Autodesk Fusion 360 part; units mm, degrees
note: some values were not read from the file. Chosen so that the rebuilt part matches the saved one: which face or edge a step refers to.
(part 2 of 2)
sketch "Sketch63" plane through (0, 0, -22) normal (0, 0, 1) x (-1, 0, 0)
  line L0 (-15, -20.0531) -> (-15, -15)
  line L1 (-15, -15) -> (-65, -15)
  line L2 (-65, -15) -> (-65, -0.5084)
  circle A0 centre (-69.7753, -0.5084) radius 4.7753
  line L3 (-65, -0.5084) -> (-65, 13.9831)
  line L4 (-65, 13.9831) -> (-82.6499, 13.9831)
  line L5 (-82.6499, 13.9831) -> (-96.6499, -0.0169)
  line L6 (-96.6499, -0.0169) -> (-96.6499, -72.0837)
  line L7 (-96.6499, -72.0837) -> (-82.6499, -86.0837)
  line L8 (-82.6499, -86.0837) -> (-65, -86.0837)
  line L9 (-65, -86.0837) -> (-65, -71.5419)
  circle A1 centre (-69.9244, -71.5419) radius 4.9244
  line L10 (-65, -71.5419) -> (-65, -57)
  line L11 (-65, -57) -> (-15, -57)
  line L12 (-15, -57) -> (-15, -52)
  line L13 (-15, -52) -> (-18, -52)
  line L14 (-18, -52) -> (-18, -20.0531)
  line L15 (-18, -20.0531) -> (-15, -20.0531)
  circle A2 centre (-85.0223, -71.5419) radius 5
  circle A3 centre (-84.8815, -0.5084) radius 5
  dimension "d174" = 10
  dimension "d175" = 10
  measures "d174" diameter of A2
  measures "d175" diameter of A3
extrude "Extrude63" cut sketch "Sketch63" against normal blind 10 contours A2 | A3 bodies 24
sketch "Sketch64" plane through (0, 0, -22) normal (0, 0, 1) x (-1, 0, 0)
  circle A0 centre (-85.0223, -71.5419) radius 5
  circle A1 centre (-84.8815, -0.5084) radius 5
  line L0 (-15, -20.0531) -> (-15, -15)
  line L1 (-15, -15) -> (-65, -15)
  line L2 (-65, -15) -> (-65, -0.5084)
  circle A2 centre (-69.7753, -0.5084) radius 4.7753
  line L3 (-65, -0.5084) -> (-65, 13.9831)
  line L4 (-65, 13.9831) -> (-82.6499, 13.9831)
  line L5 (-82.6499, 13.9831) -> (-96.6499, -0.0169)
  line L6 (-96.6499, -0.0169) -> (-96.6499, -72.0837)
  line L7 (-96.6499, -72.0837) -> (-82.6499, -86.0837)
  line L8 (-82.6499, -86.0837) -> (-65, -86.0837)
  line L9 (-65, -86.0837) -> (-65, -71.5419)
  circle A3 centre (-69.9244, -71.5419) radius 4.9244
  line L10 (-65, -71.5419) -> (-65, -57)
  line L11 (-65, -57) -> (-15, -57)
  line L12 (-15, -57) -> (-15, -52)
  line L13 (-15, -52) -> (-18, -52)
  line L14 (-18, -52) -> (-18, -20.0531)
  line L15 (-18, -20.0531) -> (-15, -20.0531)
  line L16 (-96.6499, -49.9799) -> (-91, -49.9799)
  line L17 (-91, -49.9799) -> (-91, -20)
  line L18 (-91, -20) -> (-96.6499, -20)
  line L19 (-96.6499, -20) -> (-96.6499, -49.9799)
  line L20 (-65, -86.0837) -> (-65, -84)
  line L21 (-65, -84) -> (-82, -84)
  line L22 (-82, -84) -> (-95, -72)
  line L23 (-95, -72) -> (-95, 0)
  line L24 (-95, 0) -> (-82, 12)
  line L25 (-82, 12) -> (-65, 12)
  constraint horizontal L16
  constraint vertical L17
  constraint horizontal L18
  constraint vertical L19
  constraint coincident L6 L16.start
  constraint coincident L8.end L9.start
  constraint coincident L9 L20.end
  constraint perpendicular L8 L20
  constraint perpendicular L20 L21
  constraint perpendicular L16 L23
  constraint coincident L3 L25.end
  constraint perpendicular L3 L25
extrude "Extrude64" add sketch "Sketch64" along normal blind 24 separate body contours L3 L4 L5 L6 L18 L23 L24 L25 | L6 L16 L18 L19 L23 | L6 L7 L8 L9 L16 L20 L21 L22 L23 makes body 26
extrude "Extrude65" cut 1 faces at (76.55, 85.3892, 2) along direction (0, 0, -1) blind 2 on bodies 26 bodies 10 26
extrude "Extrude66" cut 1 faces at (76.55, 85.3892, 0) along direction (0, 0, -1) blind 1 on bodies 26 bodies 26
sketch "Sketch65" plane through (0, 0, 6.5) normal (0, 0, 1) x (-1, 0, 0)
  line L0 (-75, -10) -> (-75, -12)
  line L1 (-75, -12) -> (-75, -60)
  line L2 (-75, -60) -> (-75, -62)
  line L3 (-75, -62) -> (-95, -62)
  line L4 (-95, -62) -> (-95, -72)
  line L5 (-95, -72) -> (-83, -84)
  line L6 (-83, -84) -> (-65, -84)
  line L7 (-65, -84) -> (-65, -57)
  line L8 (-65, -57) -> (-26, -57)
  line L9 (-26, -57) -> (-26, -15)
  line L10 (-26, -15) -> (-65, -15)
  line L11 (-65, -15) -> (-65, 12)
  line L12 (-65, 12) -> (-83, 12)
  line L13 (-83, 12) -> (-95, 0)
  line L14 (-95, 0) -> (-95, -10)
  line L15 (-95, -10) -> (-75, -10)
  circle A0 centre (-69.7753, -0.5084) radius 1.5
  circle A1 centre (-69.9244, -71.5419) radius 1.5
  circle A2 centre (-90, -70) radius 2.5
  circle A3 centre (-90, -2) radius 2.5
  circle A4 centre (-81, -70) radius 2
  circle A5 centre (-81, -2) radius 2
  dimension "d184" = 5
  dimension "d185" = 5
  dimension "d186" = 4
  dimension "d187" = 4
  measures "d184" diameter of A2
  measures "d185" diameter of A3
  measures "d186" diameter of A4
  measures "d187" diameter of A5
extrude "Extrude67" cut sketch "Sketch65" against normal blind 3 contours A2 | A3 | A4 | A5 bodies 25
sketch "Sketch66" plane through (0, 0, -1) normal (0, 0, 1) x (-1, 0, 0)
  line L0 (-82, 12) -> (-65, 12)
  line L1 (-65, 12) -> (-65, 13.9831)
  line L2 (-65, 13.9831) -> (-82.6499, 13.9831)
  line L3 (-82.6499, 13.9831) -> (-96.6499, -0.0169)
  line L4 (-96.6499, -0.0169) -> (-96.6499, -72.0837)
  line L5 (-96.6499, -72.0837) -> (-82.6499, -86.0837)
  line L6 (-82.6499, -86.0837) -> (-65, -86.0837)
  line L7 (-65, -86.0837) -> (-65, -84)
  line L8 (-65, -84) -> (-82, -84)
  line L9 (-82, -84) -> (-95, -72)
  line L10 (-95, -72) -> (-95, 0)
  line L11 (-95, 0) -> (-82, 12)
  line L12 (-96.6499, -60.0117) -> (-95, -60.0117)
  line L13 (-95, -60.0117) -> (-95, -12)
  line L14 (-95, -12) -> (-96.6499, -12)
  line L15 (-96.6499, -12) -> (-96.6499, -60.0117)
  constraint horizontal L12
  constraint vertical L13
  constraint horizontal L14
  constraint vertical L15
  constraint coincident L10 L13.end
  constraint coincident L4 L12.start
extrude "Extrude68" add sketch "Sketch66" along normal blind 5 contours L0 L1 L2 L3 L4 L10 L11 L14 | L4 L5 L6 L7 L8 L9 L10 L12 bodies 26
sketch "Sketch67" plane through (0, 0, -22) normal (0, 0, 1) x (-1, 0, 0)
  circle A0 centre (-85.0223, -71.5419) radius 5
  circle A1 centre (-84.8815, -0.5084) radius 5
  line L0 (-15, -20.0531) -> (-15, -15)
  line L1 (-15, -15) -> (-65, -15)
  line L2 (-65, -15) -> (-65, -0.5084)
  circle A2 centre (-69.7753, -0.5084) radius 4.7753
  line L3 (-65, -0.5084) -> (-65, 13.9831)
  line L4 (-65, 13.9831) -> (-82.6499, 13.9831)
  line L5 (-82.6499, 13.9831) -> (-96.6499, -0.0169)
  line L6 (-96.6499, -0.0169) -> (-96.6499, -72.0837)
  line L7 (-96.6499, -72.0837) -> (-82.6499, -86.0837)
  line L8 (-82.6499, -86.0837) -> (-65, -86.0837)
  line L9 (-65, -86.0837) -> (-65, -71.5419)
  circle A3 centre (-69.9244, -71.5419) radius 4.9244
  line L10 (-65, -71.5419) -> (-65, -57)
  line L11 (-65, -57) -> (-15, -57)
  line L12 (-15, -57) -> (-15, -52)
  line L13 (-15, -52) -> (-18, -52)
  line L14 (-18, -52) -> (-18, -20.0531)
  line L15 (-18, -20.0531) -> (-15, -20.0531)
  line L16 (-95, -50) -> (-90, -50)
  line L17 (-90, -50) -> (-90, -20)
  line L18 (-90, -20) -> (-95, -20)
  line L19 (-95, -20) -> (-95, -50)
  constraint horizontal L16
  constraint vertical L17
  constraint horizontal L18
  constraint vertical L19
extrude "Extrude69" add sketch "Sketch67" along normal blind 10 contours L16 L17 L18 L19 bodies 24
sketch "Sketch68" plane through (95, 0, 0) normal (1, 0, 0) x (0, 1, 0)
  line L0 (20, -22) -> (50, -22)
  line L1 (50, -22) -> (50, -12)
  line L2 (50, -12) -> (20, -12)
  line L3 (20, -12) -> (20, -22)
  circle A0 centre (45, -17) radius 1.5
  circle A1 centre (25, -17) radius 1.5
  dimension "d194" = 3
  dimension "d195" = 3
  measures "d194" diameter of A0
  measures "d195" diameter of A1
extrude "Extrude70" cut sketch "Sketch68" against normal blind 10 contours A0 | A1 bodies 24
extrude "Extrude71" cut sketch "Sketch68" along normal blind 4 contours A0 | A1 bodies 26
extrude "Extrude72" add 2 faces at (76.55, 85.3892, 4) (76.55, -13.3221, 4) along direction (0, 0, 1) blind 1 on bodies 26 bodies 26
extrude "Extrude73" cut 2 faces at (96, 49.7337, 4.7398) (96, 25.3431, 3.7629) along direction (-1, 0, 0) blind 12 on bodies 10 bodies 10
extrude "Extrude74" cut 2 faces at (95, 24.4418, 1.8385) (95, 49.4418, 1.8385) along direction (-1, 0, 0) blind 11 on bodies 10 bodies 10
sketch "Sketch69" plane through (84, 0, 0) normal (1, 0, 0) x (0, 1, 0)
  line L0 (58.5, 19) -> (13.5, 19)
  line L1 (13.5, 19) -> (13.5, -1)
  line L2 (13.5, -1) -> (58.5, -1)
  line L3 (58.5, -1) -> (58.5, 19)
  circle A0 centre (49.9081, 9) radius 8
  circle A1 centre (21.9658, 9) radius 8
  dimension "d206" = 16
  dimension "d207" = 16
  measures "d206" diameter of A0
  measures "d207" diameter of A1
extrude "Extrude75" add sketch "Sketch69" along normal blind 12 contours A0 | A1 bodies 10
sketch "Sketch70" plane through (95, 0, 0) normal (1, 0, 0) x (0, 1, 0)
  circle A0 centre (45, -17) radius 1.5
  circle A1 centre (25, -17) radius 1.5
  line L0 (20, -22) -> (50, -22)
  line L1 (50, -22) -> (50, -12)
  line L2 (50, -12) -> (20, -12)
  line L3 (20, -12) -> (20, -22)
  line L4 (50, -12) -> (58.5, -1)
  line L5 (58.5, -1) -> (58.5, 19)
  line L6 (58.5, 19) -> (13.5, 19)
  line L7 (13.5, 19) -> (13.5, -1)
  line L8 (13.5, -1) -> (20, -12)
  constraint coincident L1.end L2.start
  constraint perpendicular L2 L5
  constraint perpendicular L5 L6
  constraint perpendicular L6 L7
  constraint coincident L2.end L3.start
sketch "Sketch71" plane through (96, 0, 0) normal (1, 0, 0) x (0, 1, 0)
  circle A0 centre (21.9658, 9) radius 8
  circle A1 centre (21.9658, 9) radius 8
  constraint concentric A0 A1
sketch "Sketch72" plane through (96, 0, 0) normal (1, 0, 0) x (0, 1, 0)
  circle A0 centre (49.9081, 9) radius 8
  circle A1 centre (49.9081, 9) radius 8
  constraint concentric A0 A1
extrude "Extrude76" add sketch "Sketch70" against normal blind 1.5 contours L2 L4 L5 L6 L7 L8 bodies 24
extrude "Extrude77" cut sketch "Sketch72" sketch "Sketch71" against normal blind 3 of sketch 2 bodies 24
sketch "Sketch73" plane through (0, 86, 0) normal (0, 1, 0) x (-1, 0, 0)
  circle A0 centre (-29.5, -11) radius 2.5
  circle A1 centre (-29.5, -11) radius 33
extrude "Extrude78" add 2 faces at (88.8333, 60.6667, 20.5) (88.8333, 11.3333, 20.5) along direction (0, 0, 1) blind 1 on bodies 25 bodies 25
sketch "Sketch74" plane through (0, 86, 0) normal (0, 1, 0) x (-1, 0, 0)
sketch "Sketch75" plane through (0, 0, -23.5) normal (0, 0, -1) x (1, 0, 0)
  circle A0 centre (85.0223, -71.5419) radius 5
  circle A1 centre (84.8815, -0.5084) radius 5
  circle A2 centre (69.9244, -71.5419) radius 1.5
  circle A3 centre (69.7753, -0.5084) radius 1.5
  line L0 (1, -20.0531) -> (18, -20.0531)
  line L1 (18, -20.0531) -> (18, -52)
  line L2 (18, -52) -> (1, -52)
  line L3 (1, -52) -> (1, -57)
  line L4 (1, -57) -> (65, -57)
  line L5 (65, -57) -> (65, -86.0837)
  line L6 (65, -86.0837) -> (82.6499, -86.0837)
  line L7 (82.6499, -86.0837) -> (96.6499, -72.0837)
  line L8 (96.6499, -72.0837) -> (96.6499, -0.0169)
  line L9 (96.6499, -0.0169) -> (82.6499, 13.9831)
  line L10 (82.6499, 13.9831) -> (65, 13.9831)
  line L11 (65, 13.9831) -> (65, -15)
  line L12 (65, -15) -> (1, -15)
  line L13 (1, -15) -> (1, -20.0531)
  circle A4 centre (75, -65) radius 5
  circle A5 centre (75, -7.0195) radius 5
  dimension "d216" = 10
  measures "d216" diameter of A5
extrude "Extrude79" add sketch "Sketch75" along normal blind 28 separate body contours A4 | A5 makes body 27 at (79.9752, 65.4978, -42.1667) makes body 28 at (79.9752, 7.5173, -42.1667)
sketch "Sketch76" plane through (0, 0, -51.5) normal (0, 0, -1) x (1, 0, 0)
  circle A0 centre (75, -65) radius 5
  circle A1 centre (75, -65) radius 1.5
  dimension "d219" = 3
  constraint concentric A0 A1
  measures "d219" diameter of A1
sketch "Sketch77" plane through (0, 0, -51.5) normal (0, 0, -1) x (1, 0, 0)
  circle A0 centre (75, -7.0195) radius 5
  circle A1 centre (75, -7.0195) radius 1.5
  dimension "d220" = 3
  constraint concentric A0 A1
  measures "d220" diameter of A1
extrude "Extrude80" cut sketch "Sketch77" sketch "Sketch76" against normal blind 40 contours A1 of sketch 2 contours A1 bodies 24 27 28
sketch "Sketch78" plane through (0, 0, -51.5) normal (0, 0, -1) x (1, 0, 0)
  circle A0 centre (75, -65) radius 1.5
  circle A1 centre (75, -65) radius 5
  line L0 (80, -75) -> (80, 0)
  line L1 (80, 0) -> (10, 0)
  line L2 (10, 0) -> (10, -65)
  line L3 (10, -65) -> (10, -68.5048)
  line L4 (10, -68.5048) -> (10, -75)
  line L5 (10, -75) -> (10, 0)
  line L6 (10, -75) -> (80, -75)
  constraint vertical L0
  constraint perpendicular L0 L1
  constraint perpendicular L1 L2
  constraint parallel L3 L4
  constraint perpendicular L1 L5
  constraint perpendicular L0 L6
extrude "Extrude81" add sketch "Sketch78" along normal blind 1.5 separate body contours A1 | L0 L1 L2 L3 L4 L5 L6 makes body 29
extrude "Extrude82" cut sketch "Sketch77" along normal blind 10 contours A1 bodies 29
chamfer "Chamfer8" distance 5 angle 45 2 edges at (80, 75, -52.25) (80, 0, -52.25) on bodies 29
hidden bodies 7 8 12 13 14 15 17 18 19 22
